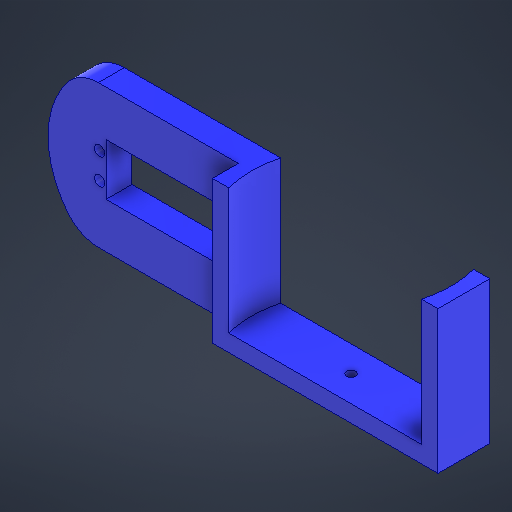
# Autodesk Inventor part: Spider_Robot_Coxa_V1
Saved by Autodesk Inventor 2026.2 (Build 302298010, 298A)
## iProperties
Created: 2026-07-24
Part Number: Spider_Robot_Coxa_V1
Material: Generic
Document SubType Name: Modeling
Designer: Entity
Mass: 50.9064 g
Surface Area: 188.873 cm^2
Volume: 50.9064 cm^3
Density: 1 g/cm^3
Appearance: Blue - Wall Paint - Glossy
Author: Entity
Autodesk Inventor part; units mm, degrees
ref_plane "YZ Plane" through (0, 0, 0) normal (1, 0, 0) x (0, 1, 0)
ref_plane "XZ Plane" through (0, 0, 0) normal (0, 1, 0) x (-1, 0, 0)
ref_plane "XY Plane" through (0, 0, 0) normal (0, 0, 1) x (1, 0, 0)
sketch "Sketch1" plane through (0, 0, 0) normal (0, 1, 0) x (-1, 0, 0)
  line L0 (43.5, -10) -> (-43.5, -10)
  line L1 (-43.5, -10) -> (-43.5, 10)
  line L2 (-43.5, 10) -> (43.5, 10)
  line L3 (43.5, 10) -> (43.5, -10)
  point P0 (0, 0)
  point P1 (-43.5, 0)
  point P2 (0, -10)
  dimension "d0" = 0
  dimension "d1" = 0
  dimension "d2" = 87
  dimension "d3" = 20
  constraints: 8 end point, 2 midpoint, 2 parallel, 1 horizontal, 1 perpendicular
  measures "d0" vertical distance of point (-43.5, 0) point (0, 0)
  measures "d1" horizontal distance of point (0, -10) point (0, 0)
  measures "d2" distance of L1.end L2.end
  measures "d3" distance of L2.end L0.start
extrude "Extrusion1" add sketch "Sketch1" along normal blind 55
sketch "Sketch2" plane through (0, 55, 0) normal (0, 1, 0) x (1, 0, 0)
  circle A0 centre (0, 0) radius 38.5
  dimension "d6" = 77
  constraints: 1 centre point, 1 coincident
  measures "d6" diameter of A0
extrude "Extrusion2" cut sketch "Sketch2" against normal blind 48.5
sketch "Sketch3" plane through (0, 0, 0) normal (0, -1, 0) x (1, 0, 0)
  line L0 (21, -10) -> (-21, -10)
  line L1 (-21, -10) -> (-21, 10)
  line L2 (-21, 10) -> (21, 10)
  line L3 (21, 10) -> (21, -10)
  line L4 (-21, 0) -> (-12, 0)
  circle A0 centre (0, 0) radius 1.75
  point P0 (0, 10)
  dimension "d11" = 42
  dimension "d12" = 20
  dimension "d17" = 3.5
  constraints: 10 end point, 2 horizontal, 2 midpoint, 2 parallel, 1 centre point, 1 coincident, 1 perpendicular
  measures "d11" distance of L0.start L0.end
  measures "d12" distance of L2.end L0.start
  measures "d17" diameter of A0
extrude "Extrusion3" cut sketch "Sketch3" against normal through all contours A0
sketch "Sketch4" plane through (-43.5, 0, -10) normal (-1, 0, 0) x (0, 0, 1)
  line L0 (0, 0) -> (20, 0) projected
  line L1 (0, 55) -> (20, 55) projected
  line L2 (0, 0) -> (10, 0)
  line L3 (10, 0) -> (10, 55)
  line L4 (10, 55) -> (0, 55)
  line L5 (0, 55) -> (0, 0)
  point P0 (10, 0)
  constraints: 8 end point, 2 parallel, 1 horizontal, 1 midpoint, 1 perpendicular
extrude "Extrusion4" add sketch "Sketch4" along normal blind 60
sketch "Sketch5" plane through (-43.5, 0, 0) normal (0, 0, 1) x (1, 0, 0)
  line L0 (0, 55) -> (0, 0) projected
  line L1 (-60, 0) -> (-60, 55) projected
  line L2 (-60, 27.5) -> (-60, 17.5)
  line L3 (-51, 17.5) -> (-9, 17.5)
  line L4 (-60, 27.5) -> (-60, 37.5)
  line L5 (-51, 37.5) -> (-9, 37.5)
  line L6 (-30, 17.5) -> (-30, 37.5)
  line L7 (-30, 17.5) -> (-51, 17.5)
  line L8 (-51, 17.5) -> (-51, 37.5)
  line L9 (-30, 37.5) -> (-9, 37.5)
  line L10 (-9, 37.5) -> (-9, 17.5)
  point P0 (43.5, 0)
  dimension "d20" = 10
  dimension "d21" = 10
  dimension "d22" = 21
  dimension "d23" = 21
  constraints: 18 end point, 4 perpendicular, 3 midpoint, 2 point on line
  measures "d20" distance of L2.start L2.end
  measures "d21" distance of L2.start L4.end
  measures "d22" distance of L3.start L6.start
  measures "d23" distance of L5.end L6.end
extrude "Extrusion5" cut sketch "Sketch5" against normal through all
sketch "Sketch6" plane through (-43.5, 0, 0) normal (0, 0, 1) x (1, 0, 0)
  line L0 (6.3214, 55) -> (-60, 55) projected
  line L1 (87, 0) -> (-60, 0) projected
  arc A0 (-60, 55) -> (-60, 0) centre (-38.3494, 27.5) ccw
  line L2 (-60, 55) -> (-60, 0) projected
  line L3 (-60, 55) -> (-60, 0)
  point P0 (43.5, 0)
  dimension "d26" = 35
  constraints: 2 end point, 2 point on circle, 1 centre point, 1 collinear
  measures "d26" radius of A0
extrude "Extrusion6" add sketch "Sketch6" against normal blind 10
fillet "Fillet1" radius 15 2 edges at (-103.5, 55, -5) (-103.5, 0, -5)
sketch "Sketch7" plane through (-43.5, 0, 0) normal (0, 0, 1) x (1, 0, 0)
  line L0 (-51, 17.5) -> (-51, 37.5) projected
  line L1 (-51, 27.5) -> (-53.5, 27.5)
  line L2 (-53.5, 27.5) -> (-53.5, 22.5)
  circle A0 centre (-53.5, 22.5) radius 2
  line L3 (-53.5, 27.5) -> (-53.5, 32.5)
  circle A1 centre (-53.5, 32.5) radius 2
  point P0 (43.5, 0)
  dimension "d30" = 2.5
  dimension "d31" = 5
  dimension "d32" = 4
  dimension "d33" = 5
  dimension "d34" = 4
  constraints: 6 end point, 2 centre point, 2 coincident, 1 horizontal, 1 midpoint, 1 perpendicular, 1 vertical
  measures "d30" distance of L1.start L1.end
  measures "d31" distance of L1.end L2.end
  measures "d32" diameter of A0
  measures "d33" distance of L1.end L3.end
  measures "d34" diameter of A1
extrude "Extrusion7" cut sketch "Sketch7" against normal through all
sketch "Sketch8" plane through (-43.5, 0, 0) normal (0, 0, 1) x (1, 0, 0)
  line L0 (-9, 37.5) -> (-9, 17.5) projected
  line L1 (-9, 27.5) -> (-6.5, 27.5)
  line L2 (-6.5, 27.5) -> (-6.5, 22.5)
  line L3 (-6.5, 27.5) -> (-6.5, 32.5)
  line L4 (0, 55) -> (-53.9619, 55) projected
  circle A0 centre (-6.5, 22.5) radius 2
  circle A1 centre (-6.5, 32.5) radius 2
  point P0 (43.5, 0)
  dimension "d37" = 2.5
  dimension "d38" = 5
  dimension "d39" = 5
  dimension "d40" = 4
  dimension "d41" = 4
  constraints: 6 end point, 2 centre point, 2 coincident, 2 perpendicular, 1 horizontal, 1 midpoint
  measures "d37" distance of L1.start L1.end
  measures "d38" distance of L1.end L2.end
  measures "d39" distance of L1.end L3.end
  measures "d40" diameter of A0
  measures "d41" diameter of A1
extrude "Extrusion8" cut sketch "Sketch8" against normal through all
body "Solid1"
